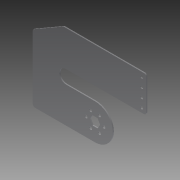
# Autodesk Inventor part: Lexan flexible Arm Mount
Saved by Autodesk Inventor 2014 (Build 180170000, 170)
## iProperties
Created: 2014-02-11
Part Number: Lexan flexible Arm Mount
Material: Polycarbonate, Clear
Document SubType Name: Modeling
Designer: Michael
Density: 1.2 g/cm^3
Appearance: Polycarbonate - Clear
Author: Michael
Autodesk Inventor part; units mm, degrees
ref_plane "YZ Plane" through (0, 0, 0) normal (1, 0, 0) x (0, 1, 0)
ref_plane "XZ Plane" through (0, 0, 0) normal (0, 1, 0) x (-1, 0, 0)
ref_plane "XY Plane" through (0, 0, 0) normal (0, 0, 1) x (1, 0, 0)
sketch "Sketch1" plane through (0, 0, 0) normal (0, 0, 1) x (1, 0, 0)
  circle A0 centre (19.05, 19.05) radius 7.9375
  line L0 (22.7162, 25.4) -> (26.3823, 19.05)
  line L1 (26.3823, 19.05) -> (22.7162, 12.7)
  line L2 (22.7162, 12.7) -> (15.3838, 12.7)
  line L3 (15.3838, 12.7) -> (11.7177, 19.05)
  line L4 (11.7177, 19.05) -> (15.3838, 25.4)
  line L5 (15.3838, 25.4) -> (22.7162, 25.4)
  circle A1 centre (6.35, 19.05) radius 2.0828
  line L6 (6.35, 19.05) -> (19.05, 19.05) construction
  circle A2 centre (12.7, 8.0515) radius 2.0828
  circle A3 centre (25.4, 8.0515) radius 2.0828
  circle A4 centre (31.75, 19.05) radius 2.0828
  circle A5 centre (25.4, 30.0485) radius 2.0828
  circle A6 centre (12.7, 30.0485) radius 2.0828
  arc A7 (19.05, -6.35) -> (19.05, 44.45) centre (19.05, 19.05) ccw
  line L7 (19.05, -6.35) -> (-69.85, -6.35)
  line L8 (19.05, 44.45) -> (-22.225, 44.45)
  line L9 (-69.85, -6.35) -> (-69.85, 88.9)
  line L10 (-25.8559, 114.3) -> (92.075, 114.3)
  line L11 (92.075, 114.3) -> (92.075, 63.5)
  line L12 (92.075, 63.5) -> (-22.225, 63.5)
  line L13 (-150.8125, 55.7276) -> (200.025, 55.7276) construction
  arc A8 (-22.225, 63.5) -> (-22.225, 44.45) centre (-22.225, 53.975) ccw
  circle A9 centre (85.725, 69.85) radius 2.0828
  circle A10 centre (85.725, 82.55) radius 2.0828
  circle A11 centre (85.725, 95.25) radius 2.0828
  circle A12 centre (85.725, 107.95) radius 2.0828
  line L14 (-22.225, 53.975) -> (-31.75, 53.975) construction
  line L15 (-69.85, 88.9) -> (-25.8559, 114.3)
  point P0 (0, 0)
  dimension "d7" = 15.875
  dimension "d8" = 12.7
  dimension "d23" = 4.1656
  dimension "d25" = 12.7
  dimension "d26" = 0
  dimension "d29" = 360
  dimension "d41" = 50.8
  dimension "d42" = 19.05
  dimension "d43" = 19.05
  dimension "d44" = 88.9
  dimension "d55" = 73.025
  dimension "d57" = 4.1656
  dimension "d58" = 6.35
  dimension "d59" = 6.35
  dimension "d62" = 12.7
  dimension "d67" = 6.35
  dimension "d68" = 36.6776
  dimension "d69" = 50.8
  dimension "d70" = 38.1
  dimension "d71" = 150
  dimension "d72" = 25.4
  dimension "d76" = 107.95
  constraints: 32 end point, 13 centre point, 5 point on circle, 4 tangent, 3 horizontal, 2 coincident, 2 parallel, 2 perpendicular, 1 vertical, 32 other
  measures "d7" diameter of A0
  measures "d8" distance between parallel lines of L5 L2
  measures "d23" diameter of A1
  measures "d25" distance of L6.end L6.start
  measures "d26" angle of L2 L6
  measures "d41" diameter of A7
  measures "d42" horizontal distance of A7.centre point (0, 0)
  measures "d43" horizontal distance of point (0, 0) A0.centre
  measures "d44" horizontal distance of A0.centre L7.end
  measures "d55" distance from line of L11 A0.centre
  measures "d57" diameter of A9
  measures "d58" distance from line of L12 A9.centre
  measures "d59" distance from line of L11 A9.centre
  measures "d62" distance of A9.centre A10.centre
  measures "d67" distance from line of L10 A12.centre
  measures "d68" distance from line of A0.centre L13
  measures "d69" vertical distance of A9.centre A0.centre
  measures "d70" distance from line of L9 L14.end
  measures "d71" angle of L10 L15
  measures "d72" distance from line of L9.end L10
  measures "d76" horizontal distance of A12.centre L12.end
extrude "Extrusion1" add sketch "Sketch1" along normal blind 1.5875 contours A0 | L7 L9 L15 L10 L11 L12 A8 L8 A7
fillet "Fillet1" radius 3.175 5 edges at (-25.8559, 114.3, 0.7937) (-69.85, 88.9, 0.7937) (92.075, 114.3, 0.7937) (92.075, 63.5, 0.7937) (-69.85, -6.35, 0.7937)
equation "\"d67\" = d58"
body "Solid1"
